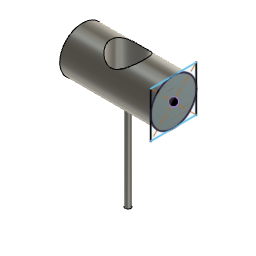
_hadle.73d7bef0-fba7-4d93-ae10-4170078bd38c (Autodesk Fusion 360 design; units mm, degrees)
Autodesk Fusion 360 part; units mm, degrees
sketch "Sketch3" plane through (0, 0, 0) normal (0, 0, 1) x (1, 0, 0)
  circle A0 centre (0, 0) radius 2.5
  circle A1 centre (0, 0) radius 2
  dimension "d8" = 5
  dimension "d9" = 4
  constraint coincident A0.centre A1.centre
  measures "d8" diameter of A0
  measures "d9" diameter of A1
extrude "Extrude1" add sketch "Sketch3" along normal blind 80 makes body 1
ref_plane "WorkPlane1" through (0, 0, 80) normal (0, 0, 1) x (1, 0, 0)
sketch "Sketch4" plane through (0, 0, 80) normal (0, 0, 1) x (1, 0, 0)
sketch "Sketch5" plane through (0, 0, 80) normal (0, 0, 1) x (-1, 0, 0)
  circle A0 centre (0, 0) radius 2
  circle A1 centre (0, 0) radius 2.5
  line L0 (-40, 20) -> (40, 20)
  line L1 (40, 20) -> (40, -20)
  line L2 (40, -20) -> (-40, -20)
  line L3 (-40, -20) -> (-40, 20)
  line L4 (-40, 20) -> (40, -20) construction
  line L5 (40, 20) -> (-40, -20) construction
  dimension "d13" = 80
  constraint horizontal L0
  constraint perpendicular L0 L1
  constraint parallel L0 L2
  constraint parallel L1 L3
  constraint coincident L4 A0.centre
  constraint coincident L5 A0.centre
  constraint coincident A0.centre A1.centre
  measures "d13" distance of L1.end L2.end
extrude "Extrude2" add sketch "Sketch5" along normal blind 40 separate body contours L0 L1 L2 L3 makes body 2
ref_plane "WorkPlane2" through (0, 0, 120) normal (0, 0, 1) x (-1, 0, 0)
sketch "Sketch6" plane through (0, 0, 120) normal (0, 0, 1) x (1, 0, 0)
ref_plane "WorkPlane3" through (40, 0, 100) normal (1, 0, 0) x (0, 1, 0)
sketch "Sketch7" plane through (40, 0, 100) normal (1, 0, 0) x (0, 1, 0)
  circle A0 centre (0, 0) radius 20
  line L0 (20, 20) -> (-20, 20)
  line L1 (-20, 20) -> (-20, -20)
  line L2 (-20, -20) -> (20, -20)
  line L3 (20, -20) -> (20, 20)
  line L4 (20, 20) -> (-20, -20) construction
  line L5 (-20, 20) -> (20, -20) construction
  dimension "d18" = 40
  dimension "d19" = 40
  constraint coincident A0.centre origin
  constraint horizontal L0
  constraint perpendicular L0 L1
  constraint parallel L0 L2
  constraint parallel L1 L3
  constraint coincident L4 A0.centre
  constraint coincident L5 A0.centre
  measures "d18" diameter of A0
  measures "d19" distance of L1.end L2.end
extrude "Extrude4" cut sketch "Sketch7" against normal blind 80 contours A0 L2 L3 | A0 L0 L3 | A0 L0 L1 | A0 L1 L2 bodies 2
extrude "Extrude3" cut sketch "Sketch7" against normal blind 80 contours A0 L0 L1 bodies 2
sketch "Sketch8" plane through (40, 0, 0) normal (1, 0, 0) x (0, 1, 0)
  circle A0 centre (0, 100) radius 20
ref_plane "WorkPlane4" through (0, 0, 120) normal (0, 0, 1) x (1, 0, 0)
sketch "Sketch9" plane through (0, 0, 120) normal (0, 0, 1) x (1, 0, 0)
  circle A0 centre (0, 0) radius 15
  dimension "d25" = 30
  constraint coincident A0.centre origin
  measures "d25" diameter of A0
extrude "Extrude5" cut sketch "Sketch9" against normal blind 25 bodies 2
